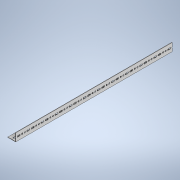
# Autodesk Inventor part: ChassisFrame
Saved by Autodesk Inventor 2020 (Build 240168000, 168)
## iProperties
Created: 2021-11-11
Part Number: ChassisFrame
Material: Generic
Document SubType Name: Modeling
Designer: 17185
Density: 1 g/cm^3
Appearance: Default
Author: 17185
Autodesk Inventor part; units mm, degrees
ref_plane "YZ Plane" through (0, 0, 0) normal (1, 0, 0) x (0, 1, 0)
ref_plane "XZ Plane" through (0, 0, 0) normal (0, 1, 0) x (-1, 0, 0)
ref_plane "XY Plane" through (0, 0, 0) normal (0, 0, 1) x (1, 0, 0)
sketch "Sketch1" plane through (0, 0, 0) normal (0, 1, 0) x (-1, 0, 0)
  line L0 (19.05, 381) -> (-19.05, 381)
  line L1 (-19.05, 381) -> (-19.05, -381)
  line L2 (-19.05, -381) -> (19.05, -381)
  line L3 (19.05, -381) -> (19.05, 381)
  line L4 (19.05, 381) -> (-19.05, -381) construction
  line L5 (-19.05, 381) -> (19.05, -381) construction
  circle A0 centre (0, 62.23) radius 3.556
  circle A1 centre (0, 6.35) radius 3.556
  line L6 (0, 381) -> (0, -381) construction
  line L7 (0, 49.53) -> (0, 40.64) construction
  line L8 (3.556, 49.53) -> (3.556, 40.64)
  line L9 (-3.556, 40.64) -> (-3.556, 49.53)
  arc A2 (3.556, 49.53) -> (-3.556, 49.53) centre (0, 49.53) ccw
  arc A3 (-3.556, 40.64) -> (3.556, 40.64) centre (0, 40.64) ccw
  line L10 (0, 27.94) -> (0, 19.05) construction
  line L11 (-3.556, 27.94) -> (-3.556, 19.05)
  line L12 (3.556, 19.05) -> (3.556, 27.94)
  arc A4 (3.556, 27.94) -> (-3.556, 27.94) centre (0, 27.94) ccw
  arc A5 (-3.556, 19.05) -> (3.556, 19.05) centre (0, 19.05) ccw
  line L13 (19.05, 68.58) -> (-6.1251, 68.58) construction
  line L14 (-6.1251, 68.58) -> (-19.05, 68.58) construction
  line L15 (19.05, 0) -> (-19.05, 0) construction
  circle A6 centre (0, -62.23) radius 3.556
  circle A7 centre (0, -6.35) radius 3.556
  line L16 (0, -49.53) -> (0, -40.64) construction
  line L17 (3.556, -49.53) -> (3.556, -40.64)
  line L18 (-3.556, -40.64) -> (-3.556, -49.53)
  arc A8 (-3.556, -49.53) -> (3.556, -49.53) centre (0, -49.53) ccw
  arc A9 (3.556, -40.64) -> (-3.556, -40.64) centre (0, -40.64) ccw
  line L19 (0, -27.94) -> (0, -19.05) construction
  line L20 (-3.556, -27.94) -> (-3.556, -19.05)
  line L21 (3.556, -19.05) -> (3.556, -27.94)
  arc A10 (-3.556, -27.94) -> (3.556, -27.94) centre (0, -27.94) ccw
  arc A11 (3.556, -19.05) -> (-3.556, -19.05) centre (0, -19.05) ccw
  line L22 (0, -109.22) -> (0, -118.11) construction
  line L23 (3.556, -118.11) -> (3.556, -109.22)
  arc A12 (3.556, -109.22) -> (-3.556, -109.22) centre (0, -109.22) ccw
  arc A13 (-3.556, -118.11) -> (3.556, -118.11) centre (0, -118.11) ccw
  circle A14 centre (0, -130.81) radius 3.556
  line L24 (-3.556, -109.22) -> (-3.556, -118.11)
  line L25 (0, -87.63) -> (0, -96.52) construction
  line L26 (-3.556, -96.52) -> (-3.556, -87.63)
  arc A15 (-3.556, -96.52) -> (3.556, -96.52) centre (0, -96.52) ccw
  arc A16 (3.556, -87.63) -> (-3.556, -87.63) centre (0, -87.63) ccw
  circle A17 centre (0, -74.93) radius 3.556
  line L27 (3.556, -87.63) -> (3.556, -96.52)
  line L28 (19.05, -137.16) -> (-19.05, -137.16) construction
  line L29 (19.05, 137.16) -> (-19.05, 137.16) construction
  line L30 (19.05, -274.32) -> (-19.05, -274.32) construction
  arc A18 (3.556, -246.38) -> (-3.556, -246.38) centre (0, -246.38) ccw
  arc A19 (-3.556, -255.27) -> (3.556, -255.27) centre (0, -255.27) ccw
  circle A20 centre (0, -267.97) radius 3.556
  line L31 (-3.556, -246.38) -> (-3.556, -255.27)
  line L32 (3.556, -255.27) -> (3.556, -246.38)
  line L33 (0, -246.38) -> (0, -255.27) construction
  line L34 (0, -224.79) -> (0, -233.68) construction
  line L35 (-3.556, -233.68) -> (-3.556, -224.79)
  circle A21 centre (0, -212.09) radius 3.556
  arc A22 (3.556, -224.79) -> (-3.556, -224.79) centre (0, -224.79) ccw
  line L36 (3.556, -224.79) -> (3.556, -233.68)
  arc A23 (-3.556, -233.68) -> (3.556, -233.68) centre (0, -233.68) ccw
  arc A24 (3.556, -177.8) -> (-3.556, -177.8) centre (0, -177.8) ccw
  arc A25 (-3.556, -165.1) -> (3.556, -165.1) centre (0, -165.1) ccw
  line L37 (0, -165.1) -> (0, -156.21) construction
  line L38 (-3.556, -165.1) -> (-3.556, -156.21)
  line L39 (3.556, -156.21) -> (3.556, -165.1)
  arc A26 (3.556, -156.21) -> (-3.556, -156.21) centre (0, -156.21) ccw
  circle A27 centre (0, -143.51) radius 3.556
  line L40 (0, -186.69) -> (0, -177.8) construction
  line L41 (-3.556, -177.8) -> (-3.556, -186.69)
  line L42 (3.556, -186.69) -> (3.556, -177.8)
  arc A28 (-3.556, -186.69) -> (3.556, -186.69) centre (0, -186.69) ccw
  circle A29 centre (0, -199.39) radius 3.556
  circle A30 centre (0, 130.81) radius 3.556
  line L43 (0, 87.63) -> (0, 96.52) construction
  line L44 (3.556, 87.63) -> (3.556, 96.52)
  line L45 (-3.556, 96.52) -> (-3.556, 87.63)
  arc A31 (-3.556, 87.63) -> (3.556, 87.63) centre (0, 87.63) ccw
  arc A32 (3.556, 96.52) -> (-3.556, 96.52) centre (0, 96.52) ccw
  line L46 (0, 109.22) -> (0, 118.11) construction
  line L47 (-3.556, 109.22) -> (-3.556, 118.11)
  line L48 (3.556, 118.11) -> (3.556, 109.22)
  arc A33 (-3.556, 109.22) -> (3.556, 109.22) centre (0, 109.22) ccw
  arc A34 (3.556, 118.11) -> (-3.556, 118.11) centre (0, 118.11) ccw
  arc A35 (3.556, 165.1) -> (-3.556, 165.1) centre (0, 165.1) ccw
  arc A36 (-3.556, 156.21) -> (3.556, 156.21) centre (0, 156.21) ccw
  circle A37 centre (0, 143.51) radius 3.556
  line L49 (-3.556, 165.1) -> (-3.556, 156.21)
  line L50 (3.556, 156.21) -> (3.556, 165.1)
  line L51 (0, 165.1) -> (0, 156.21) construction
  line L52 (0, 186.69) -> (0, 177.8) construction
  line L53 (-3.556, 177.8) -> (-3.556, 186.69)
  circle A38 centre (0, 199.39) radius 3.556
  arc A39 (3.556, 186.69) -> (-3.556, 186.69) centre (0, 186.69) ccw
  line L54 (3.556, 186.69) -> (3.556, 177.8)
  arc A40 (-3.556, 177.8) -> (3.556, 177.8) centre (0, 177.8) ccw
  arc A41 (3.556, 233.68) -> (-3.556, 233.68) centre (0, 233.68) ccw
  arc A42 (-3.556, 246.38) -> (3.556, 246.38) centre (0, 246.38) ccw
  line L55 (0, 246.38) -> (0, 255.27) construction
  line L56 (-3.556, 246.38) -> (-3.556, 255.27)
  line L57 (3.556, 255.27) -> (3.556, 246.38)
  arc A43 (3.556, 255.27) -> (-3.556, 255.27) centre (0, 255.27) ccw
  circle A44 centre (0, 267.97) radius 3.556
  line L58 (0, 224.79) -> (0, 233.68) construction
  line L59 (-3.556, 233.68) -> (-3.556, 224.79)
  line L60 (3.556, 224.79) -> (3.556, 233.68)
  arc A45 (-3.556, 224.79) -> (3.556, 224.79) centre (0, 224.79) ccw
  circle A46 centre (0, 212.09) radius 3.556
  arc A47 (3.556, 392.43) -> (-3.556, 392.43) centre (0, 392.43) ccw
  line L61 (0, 383.54) -> (0, 392.43) construction
  line L62 (-3.556, 383.54) -> (-3.556, 392.43)
  line L63 (3.556, 392.43) -> (3.556, 383.54)
  arc A48 (-3.556, 383.54) -> (3.556, 383.54) centre (0, 383.54) ccw
  arc A49 (3.556, 370.84) -> (-3.556, 370.84) centre (0, 370.84) ccw
  line L64 (0, 361.95) -> (0, 370.84) construction
  line L65 (-3.556, 370.84) -> (-3.556, 361.95)
  line L66 (3.556, 361.95) -> (3.556, 370.84)
  arc A50 (-3.556, 361.95) -> (3.556, 361.95) centre (0, 361.95) ccw
  circle A51 centre (0, 349.25) radius 3.556
  circle A52 centre (0, 336.55) radius 3.556
  arc A53 (3.556, 323.85) -> (-3.556, 323.85) centre (0, 323.85) ccw
  line L67 (0, 323.85) -> (0, 314.96) construction
  line L68 (-3.556, 314.96) -> (-3.556, 323.85)
  line L69 (3.556, 323.85) -> (3.556, 314.96)
  arc A54 (-3.556, 314.96) -> (3.556, 314.96) centre (0, 314.96) ccw
  arc A55 (3.556, 302.26) -> (-3.556, 302.26) centre (0, 302.26) ccw
  line L70 (-3.556, 302.26) -> (-3.556, 293.37)
  line L71 (3.556, 293.37) -> (3.556, 302.26)
  line L72 (0, 302.26) -> (0, 293.37) construction
  arc A56 (-3.556, 293.37) -> (3.556, 293.37) centre (0, 293.37) ccw
  circle A57 centre (0, 280.67) radius 3.556
  line L73 (19.05, -929.64) -> (-19.05, -167.64) construction
  line L74 (-19.05, -929.64) -> (19.05, -167.64) construction
  line L75 (0, -929.64) -> (0, -167.64) construction
  circle A58 centre (0, -280.67) radius 3.556
  arc A59 (3.556, -293.37) -> (-3.556, -293.37) centre (0, -293.37) ccw
  line L76 (0, -302.26) -> (0, -293.37) construction
  line L77 (-3.556, -302.26) -> (-3.556, -293.37)
  line L78 (3.556, -293.37) -> (3.556, -302.26)
  arc A60 (-3.556, -302.26) -> (3.556, -302.26) centre (0, -302.26) ccw
  arc A61 (3.556, -314.96) -> (-3.556, -314.96) centre (0, -314.96) ccw
  line L79 (0, -323.85) -> (0, -314.96) construction
  line L80 (-3.556, -314.96) -> (-3.556, -323.85)
  line L81 (3.556, -323.85) -> (3.556, -314.96)
  arc A62 (-3.556, -323.85) -> (3.556, -323.85) centre (0, -323.85) ccw
  circle A63 centre (0, -336.55) radius 3.556
  circle A64 centre (0, -349.25) radius 3.556
  arc A65 (3.556, -361.95) -> (-3.556, -361.95) centre (0, -361.95) ccw
  line L82 (0, -361.95) -> (0, -370.84) construction
  line L83 (-3.556, -370.84) -> (-3.556, -361.95)
  line L84 (3.556, -361.95) -> (3.556, -370.84)
  arc A66 (-3.556, -370.84) -> (3.556, -370.84) centre (0, -370.84) ccw
  arc A67 (3.556, -383.54) -> (-3.556, -383.54) centre (0, -383.54) ccw
  line L85 (-3.556, -383.54) -> (-3.556, -392.43)
  line L86 (3.556, -392.43) -> (3.556, -383.54)
  line L87 (0, -383.54) -> (0, -392.43) construction
  arc A68 (-3.556, -392.43) -> (3.556, -392.43) centre (0, -392.43) ccw
  point P0 (0, 0)
  point P1 (0, 45.085)
  point P2 (0, 23.495)
  point P3 (0, -45.085)
  point P4 (0, -23.495)
  point P5 (-6.1251, -68.58)
  point P6 (0, -113.665)
  point P7 (0, -92.075)
  point P8 (0, -274.32)
  point P9 (0, -250.825)
  point P10 (0, -229.235)
  point P11 (0, -160.655)
  point P12 (-6.1251, -205.74)
  point P13 (0, -182.245)
  point P14 (0, 137.16)
  point P15 (0, 74.93)
  point P16 (0, 92.075)
  point P17 (0, 113.665)
  point P18 (0, 160.655)
  point P19 (0, 182.245)
  point P20 (0, 250.825)
  point P21 (-6.1251, 205.74)
  point P22 (0, 229.235)
  point P23 (0, 387.985)
  point P24 (0, 366.395)
  point P25 (-6.1251, 342.9)
  point P26 (0, 319.405)
  point P27 (0, 297.815)
  point P28 (0, -297.815)
  point P29 (0, -319.405)
  point P30 (-6.1251, -342.9)
  point P31 (0, -366.395)
  point P32 (0, -387.985)
  point P33 (-2.4887, -381)
  point P34 (2.4887, -381)
  point P35 (2.4887, 381)
  point P36 (-2.4887, 381)
  dimension "d1" = 762
  dimension "d3" = 7.112
  dimension "d6" = 7.112
  dimension "d9" = 3.556
  dimension "d10" = 3.556
  dimension "d11" = 6.35
  dimension "d12" = 12.7
  dimension "d13" = 8.89
  dimension "d14" = 8.89
  dimension "d15" = 12.7
  dimension "d16" = 12.7
  dimension "d26" = 6.35
  dimension "d29" = 6.35
  constraints: 224 end point, 173 symmetric about line, 96 point on circle, 69 centre point, 11 point on line, 8 midpoint, 8 tangent, 4 parallel, 3 perpendicular, 2 horizontal, 57 other
  measures "d1" distance of L0.end L1.end
  measures "d3" diameter of A1
  measures "d6" diameter of A0
  measures "d9" radius of A5
  measures "d10" radius of A3
  measures "d11" distance of A1.centre point (0, 0)
  measures "d12" distance of L10.end A1.centre
  measures "d13" distance of L10.start L10.end
  measures "d14" distance of L7.start L7.end
  measures "d15" distance of L10.start L7.end
  measures "d16" distance of L7.start A0.centre
  measures "d26" distance from line of A0.centre L13
  measures "d29" distance from line of L28 A14.centre
extrude "Extrusion1" add sketch "Sketch1" along normal blind 1.9844 contours L3 L2 A67 L1 L0 A48
sketch "Sketch5" plane through (19.05, 0, 381) normal (1, 0, 0) x (0, 0, -1)
  line L0 (0.0028, 0.1675) -> (762.0028, 0.1675)
  line L1 (762.0028, 0.1675) -> (762.0028, 38.2675)
  line L2 (762.0028, 38.2675) -> (0.0028, 38.2675)
  line L3 (0.0028, 38.2675) -> (0.0028, 0.1675)
  line L4 (381, 0) -> (381.0028, 38.2675) construction
  circle A0 centre (374.6514, 18.721) radius 3.556
  line L5 (361.9514, 18.7047) -> (353.0614, 18.6933) construction
  line L6 (361.9468, 22.2607) -> (353.0568, 22.2493)
  line L7 (353.066, 15.1373) -> (361.9559, 15.1487)
  arc A1 (361.9559, 15.1487) -> (361.9468, 22.2607) centre (361.9514, 18.7047) ccw
  arc A2 (353.0568, 22.2493) -> (353.066, 15.1373) centre (353.0614, 18.6933) ccw
  line L8 (0, 0) -> (762, 0) construction
  line L9 (346.7114, 38.2675) -> (346.7114, 0) construction
  circle A3 centre (318.7714, 18.721) radius 3.556
  line L10 (331.4714, 18.7047) -> (340.3614, 18.6933) construction
  line L11 (331.476, 22.2607) -> (340.366, 22.2493)
  line L12 (340.3568, 15.1373) -> (331.4668, 15.1487)
  arc A4 (331.476, 22.2607) -> (331.4668, 15.1487) centre (331.4714, 18.7047) ccw
  arc A5 (340.3568, 15.1373) -> (340.366, 22.2493) centre (340.3614, 18.6933) ccw
  line L13 (312.4214, 38.2675) -> (312.4214, 0) construction
  circle A6 centre (250.1914, 18.721) radius 3.556
  line L14 (262.8914, 18.7047) -> (271.7814, 18.6933) construction
  line L15 (262.896, 22.2607) -> (271.786, 22.2493)
  line L16 (271.7769, 15.1373) -> (262.8869, 15.1487)
  arc A7 (262.896, 22.2607) -> (262.8869, 15.1487) centre (262.8914, 18.7047) ccw
  arc A8 (271.7769, 15.1373) -> (271.786, 22.2493) centre (271.7814, 18.6933) ccw
  line L17 (293.3714, 18.7047) -> (284.4814, 18.6933) construction
  line L18 (284.486, 15.1373) -> (293.376, 15.1487)
  arc A9 (284.4769, 22.2493) -> (284.486, 15.1373) centre (284.4814, 18.6933) ccw
  circle A10 centre (306.0714, 18.721) radius 3.556
  arc A11 (293.376, 15.1487) -> (293.3668, 22.2607) centre (293.3714, 18.7047) ccw
  line L19 (293.3668, 22.2607) -> (284.4769, 22.2493)
  line L20 (243.8414, 38.2675) -> (243.8414, 0) construction
  circle A12 centre (113.0314, 18.721) radius 3.556
  line L21 (125.7314, 18.7047) -> (134.6214, 18.6933) construction
  line L22 (125.736, 22.2607) -> (134.626, 22.2493)
  line L23 (134.6169, 15.1373) -> (125.7269, 15.1487)
  arc A13 (125.736, 22.2607) -> (125.7269, 15.1487) centre (125.7314, 18.7047) ccw
  arc A14 (134.6169, 15.1373) -> (134.626, 22.2493) centre (134.6214, 18.6933) ccw
  line L24 (156.2114, 18.7047) -> (147.3214, 18.6933) construction
  line L25 (147.326, 15.1373) -> (156.216, 15.1487)
  arc A15 (147.3169, 22.2493) -> (147.326, 15.1373) centre (147.3214, 18.6933) ccw
  circle A16 centre (168.9114, 18.721) radius 3.556
  arc A17 (156.216, 15.1487) -> (156.2069, 22.2607) centre (156.2114, 18.7047) ccw
  line L26 (156.2069, 22.2607) -> (147.3169, 22.2493)
  arc A18 (194.316, 22.2607) -> (194.3069, 15.1487) centre (194.3114, 18.7047) ccw
  line L27 (194.3114, 18.7047) -> (203.2014, 18.6933) construction
  line L28 (194.316, 22.2607) -> (203.206, 22.2493)
  arc A19 (203.1969, 15.1373) -> (203.206, 22.2493) centre (203.2014, 18.6933) ccw
  arc A20 (215.8969, 22.2493) -> (215.906, 15.1373) centre (215.9014, 18.6933) ccw
  line L29 (224.7869, 22.2607) -> (215.8969, 22.2493)
  line L30 (215.906, 15.1373) -> (224.796, 15.1487)
  arc A21 (224.796, 15.1487) -> (224.7869, 22.2607) centre (224.7914, 18.7047) ccw
  circle A22 centre (237.4914, 18.721) radius 3.556
  circle A23 centre (181.6114, 18.721) radius 3.556
  line L31 (224.7914, 18.7047) -> (215.9014, 18.6933) construction
  line L32 (203.1969, 15.1373) -> (194.3069, 15.1487)
  line L33 (106.6814, 38.2675) -> (106.6814, 0) construction
  arc A24 (87.636, 15.1487) -> (87.6269, 22.2607) centre (87.6314, 18.7047) ccw
  line L34 (87.6314, 18.7047) -> (78.7415, 18.6933) construction
  line L35 (78.746, 15.1373) -> (87.636, 15.1487)
  arc A25 (78.7369, 22.2493) -> (78.746, 15.1373) centre (78.7415, 18.6933) ccw
  arc A26 (66.0369, 15.1373) -> (66.046, 22.2493) centre (66.0415, 18.6933) ccw
  line L36 (57.1515, 18.7047) -> (66.0415, 18.6933) construction
  arc A27 (57.156, 22.2607) -> (57.1469, 15.1487) centre (57.1515, 18.7047) ccw
  circle A28 centre (100.3314, 18.721) radius 3.556
  line L37 (87.6269, 22.2607) -> (78.7369, 22.2493)
  circle A29 centre (44.4515, 18.721) radius 3.556
  line L38 (57.156, 22.2607) -> (66.046, 22.2493)
  line L39 (66.0369, 15.1373) -> (57.1469, 15.1487)
  circle A30 centre (31.7515, 18.721) radius 3.556
  arc A31 (19.056, 15.1487) -> (19.0469, 22.2607) centre (19.0515, 18.7047) ccw
  line L40 (19.0469, 22.2607) -> (10.1569, 22.2493)
  line L41 (19.0515, 18.7047) -> (10.1615, 18.6933) construction
  line L42 (10.166, 15.1373) -> (19.056, 15.1487)
  arc A32 (10.1569, 22.2493) -> (10.166, 15.1373) centre (10.1615, 18.6933) ccw
  arc A33 (-2.5431, 15.1373) -> (-2.534, 22.2493) centre (-2.5385, 18.6933) ccw
  line L43 (-11.424, 22.2607) -> (-2.534, 22.2493)
  line L44 (-11.4285, 18.7047) -> (-2.5385, 18.6933) construction
  line L45 (-2.5431, 15.1373) -> (-11.4331, 15.1487)
  arc A34 (-11.424, 22.2607) -> (-11.4331, 15.1487) centre (-11.4285, 18.7047) ccw
  circle A35 centre (387.3514, 18.7201) radius 3.556
  line L46 (400.0514, 18.7019) -> (408.9414, 18.6892) construction
  line L47 (400.0565, 22.2579) -> (408.9465, 22.2452)
  line L48 (408.9363, 15.1332) -> (400.0463, 15.1459)
  arc A36 (400.0565, 22.2579) -> (400.0463, 15.1459) centre (400.0514, 18.7019) ccw
  arc A37 (408.9363, 15.1332) -> (408.9465, 22.2452) centre (408.9414, 18.6892) ccw
  line L49 (430.5314, 18.6974) -> (421.6414, 18.6873) construction
  line L50 (421.6454, 15.1313) -> (430.5354, 15.1414)
  arc A38 (421.6373, 22.2433) -> (421.6454, 15.1313) centre (421.6414, 18.6873) ccw
  circle A39 centre (443.2314, 18.7118) radius 3.556
  arc A40 (430.5354, 15.1414) -> (430.5273, 22.2534) centre (430.5314, 18.6974) ccw
  line L51 (430.5273, 22.2534) -> (421.6373, 22.2433)
  arc A41 (468.6365, 22.2477) -> (468.6263, 15.1357) centre (468.6314, 18.6917) ccw
  line L52 (468.6314, 18.6917) -> (477.5214, 18.679) construction
  line L53 (468.6365, 22.2477) -> (477.5264, 22.235)
  arc A42 (477.5163, 15.123) -> (477.5264, 22.235) centre (477.5214, 18.679) ccw
  arc A43 (490.2173, 22.2331) -> (490.2254, 15.1211) centre (490.2214, 18.6771) ccw
  line L54 (499.1073, 22.2432) -> (490.2173, 22.2331)
  line L55 (490.2254, 15.1211) -> (499.1154, 15.1312)
  arc A44 (499.1154, 15.1312) -> (499.1073, 22.2432) centre (499.1114, 18.6872) ccw
  circle A45 centre (511.8114, 18.7016) radius 3.556
  circle A46 centre (455.9314, 18.7099) radius 3.556
  line L56 (499.1114, 18.6872) -> (490.2214, 18.6771) construction
  line L57 (477.5163, 15.123) -> (468.6263, 15.1357)
  arc A47 (636.2754, 15.1109) -> (636.2673, 22.2229) centre (636.2713, 18.6669) ccw
  line L58 (636.2713, 18.6669) -> (627.3813, 18.6568) construction
  line L59 (627.3854, 15.1008) -> (636.2754, 15.1109)
  arc A48 (627.3773, 22.2128) -> (627.3854, 15.1008) centre (627.3813, 18.6568) ccw
  arc A49 (614.6762, 15.1027) -> (614.6864, 22.2147) centre (614.6813, 18.6587) ccw
  line L60 (605.7913, 18.6714) -> (614.6813, 18.6587) construction
  arc A50 (605.7964, 22.2274) -> (605.7863, 15.1154) centre (605.7913, 18.6714) ccw
  circle A51 centre (648.9713, 18.6813) radius 3.556
  line L61 (636.2673, 22.2229) -> (627.3773, 22.2128)
  circle A52 centre (593.0913, 18.6896) radius 3.556
  line L62 (605.7964, 22.2274) -> (614.6864, 22.2147)
  line L63 (614.6762, 15.1027) -> (605.7863, 15.1154)
  circle A53 centre (580.3913, 18.6914) radius 3.556
  arc A54 (567.6954, 15.1211) -> (567.6873, 22.233) centre (567.6913, 18.6771) ccw
  line L64 (567.6873, 22.233) -> (558.7973, 22.223)
  line L65 (567.6913, 18.6771) -> (558.8013, 18.667) construction
  line L66 (558.8054, 15.111) -> (567.6954, 15.1211)
  arc A55 (558.7973, 22.223) -> (558.8054, 15.111) centre (558.8013, 18.667) ccw
  arc A56 (546.0963, 15.1129) -> (546.1064, 22.2249) centre (546.1013, 18.6689) ccw
  line L67 (537.2164, 22.2376) -> (546.1064, 22.2249)
  line L68 (537.2114, 18.6816) -> (546.1013, 18.6689) construction
  line L69 (546.0963, 15.1129) -> (537.2063, 15.1256)
  arc A57 (537.2164, 22.2376) -> (537.2063, 15.1256) centre (537.2114, 18.6816) ccw
  circle A58 centre (524.5114, 18.6997) radius 3.556
  arc A59 (773.4353, 15.0905) -> (773.4273, 22.2025) centre (773.4313, 18.6465) ccw
  line L70 (764.5453, 15.0805) -> (773.4353, 15.0905)
  line L71 (773.4313, 18.6465) -> (764.5413, 18.6365) construction
  line L72 (773.4273, 22.2025) -> (764.5373, 22.1925)
  arc A60 (764.5373, 22.1925) -> (764.5453, 15.0805) centre (764.5413, 18.6365) ccw
  arc A61 (674.3764, 22.2172) -> (674.3662, 15.1052) centre (674.3713, 18.6612) ccw
  line L73 (674.3713, 18.6612) -> (683.2613, 18.6485) construction
  line L74 (683.2562, 15.0925) -> (674.3662, 15.1052)
  arc A62 (683.2562, 15.0925) -> (683.2664, 22.2045) centre (683.2613, 18.6485) ccw
  arc A63 (695.9573, 22.2026) -> (695.9653, 15.0906) centre (695.9613, 18.6466) ccw
  line L75 (704.8513, 18.6567) -> (695.9613, 18.6466) construction
  arc A64 (704.8553, 15.1007) -> (704.8473, 22.2127) centre (704.8513, 18.6567) ccw
  circle A65 centre (661.6713, 18.6794) radius 3.556
  line L76 (674.3764, 22.2172) -> (683.2664, 22.2045)
  line L77 (695.9653, 15.0906) -> (704.8553, 15.1007)
  line L78 (704.8473, 22.2127) -> (695.9573, 22.2026)
  line L79 (742.9564, 22.2071) -> (751.8464, 22.1943)
  line L80 (742.9513, 18.6511) -> (751.8413, 18.6384) construction
  line L81 (751.8362, 15.0824) -> (742.9462, 15.0951)
  arc A66 (742.9564, 22.2071) -> (742.9462, 15.0951) centre (742.9513, 18.6511) ccw
  circle A67 centre (730.2513, 18.6692) radius 3.556
  circle A68 centre (717.5513, 18.6711) radius 3.556
  arc A69 (751.8362, 15.0824) -> (751.8464, 22.1943) centre (751.8413, 18.6384) ccw
  point P0 (357.5064, 18.699)
  point P1 (335.9164, 18.699)
  point P2 (267.3364, 18.699)
  point P3 (288.9264, 18.699)
  point P4 (130.1764, 18.699)
  point P5 (151.7664, 18.699)
  point P6 (198.7564, 18.699)
  point P7 (220.3464, 18.699)
  point P8 (761.9999, 18.1843)
  point P9 (83.1865, 18.699)
  point P10 (61.5965, 18.699)
  point P11 (14.6065, 18.699)
  point P12 (-6.9835, 18.699)
  point P13 (404.4964, 18.6956)
  point P14 (426.0864, 18.6924)
  point P15 (473.0764, 18.6854)
  point P16 (494.6664, 18.6822)
  point P17 (631.8263, 18.6618)
  point P18 (610.2363, 18.665)
  point P19 (563.2463, 18.672)
  point P20 (541.6564, 18.6752)
  point P21 (768.9863, 18.6415)
  point P22 (678.8163, 18.6549)
  point P23 (700.4063, 18.6517)
  point P24 (747.3963, 18.6447)
  point P25 (0.0028, 21.1806)
  point P26 (0.0028, 16.2061)
  point P27 (762.0028, 16.1462)
  point P28 (762.0028, 21.1267)
  dimension "d61" = 762
  dimension "d62" = 38.1
  dimension "d63" = 7.112
  dimension "d64" = 8.89
  dimension "d65" = 7.112
  dimension "d66" = 6.35
  dimension "d67" = 12.7
  dimension "d72" = 6.35
  dimension "d73" = 6.35
  dimension "d74" = 6.35
  dimension "d75" = 6.35
  constraints: 210 end point, 182 symmetric about line, 96 point on circle, 70 centre point, 8 point on line, 4 tangent, 3 parallel, 3 perpendicular, 2 midpoint, 2 vertical, 1 horizontal, 67 other
  measures "d61" distance of L2.end L1.end
  measures "d62" distance of L0.end L1.end
  measures "d63" diameter of A0
  measures "d64" distance of L5.start L5.end
  measures "d65" diameter of A2
  measures "d66" distance from line of L4 A0.centre
  measures "d67" distance of A0.centre L5.start
  measures "d72" distance from line of L9 L5.end
  measures "d73" distance from line of L13 A3.centre
  measures "d74" distance from line of L20 A6.centre
  measures "d75" distance from line of L33 A12.centre
extrude "Extrusion2" add sketch "Sketch5" against normal blind 1.9844 contours L3 A33 L2 L1 A60 L0
equation "\"d6\" = d3"
equation "\"d9\" = 0.5 * d3"
equation "\"d10\" = d9"
equation "\"d14\" = d13"
equation "\"d15\" = d12"
equation "\"d16\" = d12"
equation "\"d65\" = d63"
equation "\"d72\" = d66"
equation "\"d73\" = d66"
equation "\"d74\" = d66"
equation "\"d75\" = d66"
body "Solid1"
